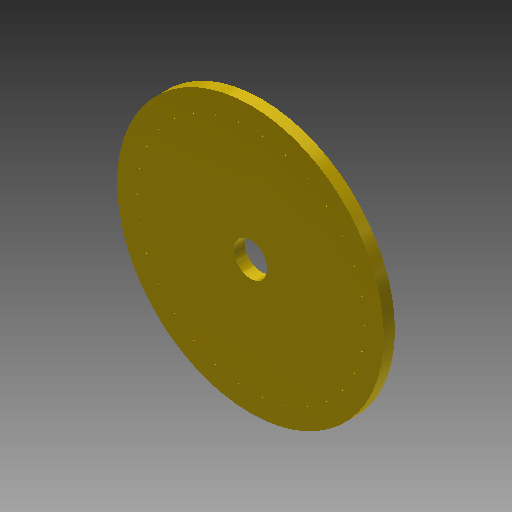
# Autodesk Inventor part: Plate between E3 and E4
Saved by Autodesk Inventor 2017 (Build 210142000, 142)
## iProperties
Created: 2009-05-07
Part Number: Plate between E3 and E4
Document SubType Name: Modeling
Designer: Serena
Material: Default
Density: 1 g/cm^3
Appearance: Glossy - Gold
Author: Serena
Autodesk Inventor part; units mm, degrees
ref_plane "YZ Plane" through (0, 0, 0) normal (1, 0, 0) x (0, 1, 0)
ref_plane "XZ Plane" through (0, 0, 0) normal (0, 1, 0) x (-1, 0, 0)
ref_plane "XY Plane" through (0, 0, 0) normal (0, 0, 1) x (1, 0, 0)
sketch "Sketch1" plane through (0, 0, 0) normal (0, 0, 1) x (1, 0, 0)
  circle A0 centre (0, 0) radius 15.25
  circle A1 centre (0, 0) radius 120.65
  dimension "d0" = 30.5
  dimension "d1" = 241.3
  constraints: 2 centre point, 1 coincident
  measures "d0" diameter of A0
  measures "d1" diameter of A1
extrude "Extrusion1" add sketch "Sketch1" along normal blind 10
sketch "Sketch2" plane through (0, 0, 0) normal (0, 1, 0) x (-1, 0, 0)
  line L0 (-120.65, 10) -> (120.65, 10) projected
  line L1 (-120.65, 0) -> (120.65, 0) projected
  line L2 (15.25, 0) -> (-15.25, 0) projected
  line L3 (-15.25, 10) -> (15.25, 10) projected
  line L4 (15.25, 0) -> (15.25, 10) projected
  line L5 (120.65, 0) -> (120.65, 10) projected
  line L6 (102.85, 10) -> (102.85, 0)
  line L7 (102.85, 10) -> (102.85, 11)
  circle A0 centre (102.85, 10.5) radius 1
  line L8 (102.85, 10) -> (102.85, 9.5)
  line L9 (102.85, 10) -> (101.984, 10)
  line L10 (102.85, 10) -> (103.716, 10)
  arc A1 (101.984, 10) -> (102.85, 9.5) centre (102.85, 10.5) ccw
  arc A2 (102.85, 9.5) -> (103.716, 10) centre (102.85, 10.5) ccw
  line L11 (15.25, 0) -> (-15.25, 0) projected
  line L12 (0, 10) -> (0, 0) construction
  dimension "d18" = 2
  dimension "d19" = 0.5
  dimension "d20" = 102.85
  constraints: 12 end point, 7 point on circle, 5 point on line, 4 concentric, 3 centre point, 3 midpoint, 1 collinear, 1 perpendicular
  measures "d18" diameter of A0
  measures "d19" distance of L6.start L8.end
  measures "d20" distance between parallel lines of L6 L12
revolve "Revolution1" cut sketch "Sketch2" angle 360 about axis through (-102.85, 0, 10) along (0, 0, -1) picked at (103.3864, 9.9436) contours L0 A0 L6
pattern_circular "Circular Pattern1" count 30 over 360 about axis through (0, 0, 0) along (0, 0, 1) of "Revolution1"
sketch "Sketch3" plane through (0, 0, 0) normal (0, 1, 0) x (-1, 0, 0)
  line L0 (15.25, 0) -> (15.25, 10) projected
  line L1 (-120.65, 10) -> (120.65, 10) projected
  line L2 (-120.65, 0) -> (120.65, 0) projected
  line L3 (120.65, 0) -> (120.65, 10) projected
  line L4 (16.75, 10) -> (16.75, 0)
  line L5 (16.75, 0) -> (16.75, -1)
  circle A0 centre (16.75, -0.5) radius 1
  line L6 (16.75, 0.5) -> (16.75, 0)
  line L7 (16.75, 0) -> (17.616, 0)
  line L8 (15.884, 0) -> (16.75, 0)
  dimension "d11" = 1.5
  dimension "d12" = 0.5
  dimension "d13" = 2
  constraints: 10 end point, 5 point on line, 3 collinear, 3 point on circle, 1 centre point, 1 midpoint, 1 perpendicular
  measures "d11" distance between parallel lines of L0 L4
  measures "d12" distance of L6.start L4.end
  measures "d13" diameter of A0
revolve "Revolution2" cut sketch "Sketch3" angle 360 about axis through (-16.75, 0, 10) along (0, 0, -1) picked at (16.2136, 0.0564) contours A0 L4 L2
pattern_circular "Circular Pattern2" count 8 over 360 about axis through (0, 0, 0) along (0, 0, 1) of "Revolution2"
body "Solid1"
